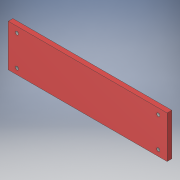
# Autodesk Inventor part: SideRail
Saved by Autodesk Inventor 2018 (Build 220112000, 112)
## iProperties
Created: 2017-12-20
Part Number: SideRail
Material: Generic
Document SubType Name: Modeling
Designer: jklei
Density: 1 g/cm^3
Appearance: Default
Author: jklei
Autodesk Inventor part; units mm, degrees
ref_plane "YZ Plane" through (0, 0, 0) normal (1, 0, 0) x (0, 1, 0)
ref_plane "XZ Plane" through (0, 0, 0) normal (0, 1, 0) x (-1, 0, 0)
ref_plane "XY Plane" through (0, 0, 0) normal (0, 0, 1) x (1, 0, 0)
sketch "Sketch1" plane through (0, 0, 0) normal (0, 0, 1) x (1, 0, 0)
  line L0 (0, 0) -> (215.9, 0)
  line L1 (215.9, 0) -> (215.9, 57.15)
  line L2 (215.9, 57.15) -> (0, 57.15)
  line L3 (0, 57.15) -> (0, 0)
  dimension "d0" = 215.9
  dimension "d1" = 57.15
  constraints: 8 end point, 2 parallel, 1 horizontal, 1 perpendicular
  measures "d0" distance of L2.end L1.end
  measures "d1" distance of L1.end L0.end
extrude "Extrusion1" add sketch "Sketch1" along normal blind 6.35
sketch "Sketch2" plane through (0, 0, 6.35) normal (0, 0, 1) x (1, 0, 0)
  line L0 (0, 57.15) -> (0, 0) projected
  line L1 (0, 57.15) -> (0, 49.15)
  line L2 (0, 49.15) -> (12, 49.15)
  circle A0 centre (12, 49.15) radius 2.1
  line L3 (0, 0) -> (0, 8)
  line L4 (0, 8) -> (12, 8)
  circle A1 centre (12, 8) radius 2.1
  line L5 (215.9, 0) -> (215.9, 57.15) projected
  line L6 (215.9, 57.15) -> (215.9, 49.15)
  line L7 (215.9, 49.15) -> (203.9, 49.15)
  circle A2 centre (203.9, 49.15) radius 2.1
  line L8 (215.9, 0) -> (215.9, 8)
  line L9 (215.9, 8) -> (203.9, 8)
  circle A3 centre (203.9, 8) radius 2.1
  dimension "d4" = 8
  dimension "d5" = 12
  dimension "d6" = 4.2
  dimension "d7" = 8
  dimension "d8" = 12
  dimension "d9" = 4.2
  dimension "d10" = 12
  dimension "d11" = 4.2
  dimension "d12" = 12
  dimension "d13" = 4.2
  constraints: 16 end point, 4 centre point, 4 coincident, 4 point on line, 3 perpendicular, 1 horizontal
  measures "d4" distance of L0.start L1.end
  measures "d5" distance of L1.end L2.end
  measures "d6" diameter of A0
  measures "d7" distance of L0.end L3.end
  measures "d8" distance of L3.end L4.end
  measures "d9" diameter of A1
  measures "d10" distance of L6.end L7.end
  measures "d11" diameter of A2
  measures "d12" distance of L8.end L9.end
  measures "d13" diameter of A3
extrude "Extrusion2" cut sketch "Sketch2" against normal through all
body "Solid1"
